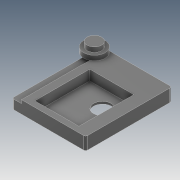
# Autodesk Inventor part: 00_XYTable_china_75_55mm
Saved by Autodesk Inventor 2022 (Build 260153000, 153)
## iProperties
Created: 2022-06-02
Part Number: 00_XYTable_china_75_55mm
Material: Generisch
Document SubType Name: Modellieren
Designer: diederichbenedict
Density: 1 g/cm^3
Appearance: Glatt - Schwarz
Author: diederichbenedict
Autodesk Inventor part; units mm, degrees
ref_plane "YZ Plane" through (0, 0, 0) normal (1, 0, 0) x (0, 1, 0)
ref_plane "XZ Plane" through (0, 0, 0) normal (0, 1, 0) x (-1, 0, 0)
ref_plane "XY Plane" through (0, 0, 0) normal (0, 0, 1) x (1, 0, 0)
sketch "Skizze1" plane through (0, 0, 0) normal (0, 1, 0) x (-1, 0, 0)
  line L0 (73.5, -90.75) -> (-73.5, -90.75)
  line L1 (-77.5, -86.75) -> (-77.5, 86.75)
  line L2 (-73.5, 90.75) -> (73.5, 90.75)
  line L3 (77.5, 86.75) -> (77.5, -86.75)
  line L4 (77.5, -90.75) -> (-77.5, 90.75) construction
  line L5 (-77.5, -90.75) -> (77.5, 90.75) construction
  arc A0 (77.5, 86.75) -> (73.5, 90.75) centre (73.5, 86.75) ccw
  arc A1 (73.5, -90.75) -> (77.5, -86.75) centre (73.5, -86.75) ccw
  arc A2 (-77.5, -86.75) -> (-73.5, -90.75) centre (-73.5, -86.75) ccw
  arc A3 (-73.5, 90.75) -> (-77.5, 86.75) centre (-73.5, 86.75) ccw
  line L6 (41.5, 78.75) -> (-51.5, 78.75)
  line L7 (-51.5, 78.75) -> (-51.5, -36.75)
  line L8 (-51.5, -36.75) -> (41.5, -36.75)
  line L9 (41.5, -36.75) -> (41.5, 78.75)
  line L10 (41.5, 78.75) -> (-51.5, -36.75) construction
  line L11 (-51.5, 78.75) -> (41.5, -36.75) construction
  point P0 (0, 0)
  point P1 (-5, 21)
  dimension "d0" = 155
  dimension "d1" = 181.5
  dimension "d2" = 4
  dimension "d3" = 12
  dimension "d4" = 26
  dimension "d5" = 54
  dimension "d6" = 36
  constraints: 24 end point, 8 point on circle, 8 point on line, 8 tangent, 4 centre point, 4 midpoint, 4 parallel, 3 equal radius, 2 horizontal, 2 perpendicular
  measures "d0" distance of L4.end L5.end
  measures "d1" distance of L5.start L4.end
  measures "d2" radius of A0
  measures "d3" distance between parallel lines of L6 L2
  measures "d4" distance between parallel lines of L7 L1
  measures "d5" distance between parallel lines of L0 L8
  measures "d6" distance between parallel lines of L3 L9
extrude "Extrusion1" add sketch "Skizze1" along normal blind 26.5
sketch "Skizze2" plane through (0, 0, 0) normal (0, -1, 0) x (1, 0, 0)
  line L0 (-73.5, 90.75) -> (73.5, 90.75) projected
  arc A0 (-73.5, 90.75) -> (-77.5, 86.75) centre (-73.5, 86.75) ccw projected
  line L1 (-77.5, -86.75) -> (-77.5, 86.75) projected
  arc A1 (-77.5, -86.75) -> (-73.5, -90.75) centre (-73.5, -86.75) ccw projected
  line L2 (73.5, -90.75) -> (-73.5, -90.75) projected
  arc A2 (73.5, -90.75) -> (77.5, -86.75) centre (73.5, -86.75) ccw projected
  line L3 (77.5, 86.75) -> (77.5, -86.75) projected
  arc A3 (77.5, 86.75) -> (73.5, 90.75) centre (73.5, 86.75) ccw projected
  line L4 (-41.5, 78.75) -> (-41.5, -36.75) projected
  line L5 (51.5, 78.75) -> (-41.5, 78.75) projected
  line L6 (51.5, -36.75) -> (51.5, 78.75) projected
  line L7 (-41.5, -36.75) -> (51.5, -36.75) projected
  circle A4 centre (22.5, 0.25) radius 18.75
  point P0 (0, 0)
  dimension "d9" = 37.5
  dimension "d11" = 90.5
  dimension "d14" = 55
  constraints: 1 centre point
  measures "d9" diameter of A4
  measures "d11" distance from line of L0 A4.centre
  measures "d14" distance from line of L3 A4.centre
extrude "Extrusion2" add sketch "Skizze2" against normal blind 5 contours L0 A3 L3 A2 L2 A1 L1 A0 | L5 L6 L7 L4
sketch "Skizze3" plane through (-73.5, 0, 90.75) normal (0, 0, 1) x (1, 0, 0)
  line L0 (-4, 0) -> (-4, 26.5) projected
  line L1 (0, 0) -> (0, 26.5) projected
  line L2 (-4, 0) -> (-4, 26.5) projected
  line L3 (-4, 26.5) -> (16, 26.5)
  line L4 (16, 26.5) -> (16, 19.2)
  line L5 (16, 19.2) -> (-4, 19.2)
  line L6 (-4, 19.2) -> (-4, 26.5)
  point P0 (73.5, 0)
  point P1 (-4, 19.2)
  dimension "d15" = 7.3
  dimension "d16" = 20
  constraints: 8 end point, 2 parallel, 1 horizontal, 1 perpendicular
  measures "d15" distance between parallel lines of L5 L3
  measures "d16" distance between parallel lines of L0 L4
extrude "Extrusion3" cut sketch "Skizze3" against normal through all
sketch "Skizze4" plane through (0, 26.5, 0) normal (0, 1, 0) x (1, 0, 0)
  line L0 (-57.5, 90.75) -> (-57.5, -90.75) projected
  line L1 (-57.5, -90.75) -> (73.5, -90.75) projected
  arc A0 (73.5, -90.75) -> (77.5, -86.75) centre (73.5, -86.75) ccw projected
  line L2 (77.5, -86.75) -> (77.5, 86.75) projected
  arc A1 (77.5, 86.75) -> (73.5, 90.75) centre (73.5, 86.75) ccw projected
  line L3 (73.5, 90.75) -> (-57.5, 90.75) projected
  line L4 (-41.5, -78.75) -> (-41.5, 36.75) projected
  line L5 (-41.5, 36.75) -> (51.5, 36.75) projected
  line L6 (51.5, 36.75) -> (51.5, -78.75) projected
  line L7 (51.5, -78.75) -> (-41.5, -78.75) projected
  arc A2 (-77.5, -86.75) -> (-73.5, -90.75) centre (-73.5, -86.75) ccw projected
  line L8 (-57.5, -90.75) -> (-73.5, -90.75) projected
  line L9 (-57.5, -90.75) -> (-57.5, 90.75) projected
  line L10 (-73.5, 90.75) -> (-57.5, 90.75) projected
  arc A3 (-73.5, 90.75) -> (-77.5, 86.75) centre (-73.5, 86.75) ccw projected
  line L11 (-77.5, -86.75) -> (-77.5, 86.75) projected
  circle A4 centre (-67.5, 72.75) radius 22.5
  point P0 (0, 0)
  dimension "d19" = 45
  dimension "d20" = 10
  dimension "d21" = 18
  constraints: 1 centre point
  measures "d19" diameter of A4
  measures "d20" distance from line of L11 A4.centre
  measures "d21" distance from line of A4.centre L3
extrude "Extrusion4" add sketch "Skizze4" along normal blind 10 contours L3 A4 L0 | L10 A3 L11 A4 L3 | L0 A4 L11 A3 L10
sketch "Skizze5" plane through (-67.5, 36.5, -72.75) normal (0, 1, 0) x (1, 0, 0)
  circle A0 centre (0, 0) radius 22.5 projected
  circle A1 centre (0, 0) radius 15
  point P0 (67.5, -72.75)
  dimension "d24" = 30
  constraints: 1 centre point, 1 coincident
  measures "d24" diameter of A1
extrude "Extrusion5" add sketch "Skizze5" along normal blind 10 contours A1
equation "\"Biegeradius\" = Stärke"
equation "\"BreiteBiegungsfreistellung\" = Stärke"
equation "\"TiefeBiegungsfreistellung\" = 0.5 * Stärke"
equation "\"GrößeEckenfreistellung\" = 4 * Stärke"
equation "\"MinimalRest\" = 2 * Stärke"
equation "\"Übergangsradius\" = Biegeradius"
equation "\"JacobiRadiusGröße\" = Biegeradius"
equation "\"Abstandsgröße\" = Stärke"
equation "\"Stärke\" = 0.5"
